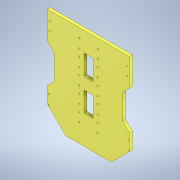
# Autodesk Inventor part: BaseCarro
Saved by Autodesk Inventor 2021 (Build 250183000, 183)
## iProperties
Created: 2021-02-05
Part Number: BaseCarro
Material: Plástico ABS
Document SubType Name: Modeling
Designer: jaime
Density: 1.06 g/cm^3
Appearance: Suave - Amarillo
Author: jaime
Autodesk Inventor part; units mm, degrees
ref_plane "YZ Plane" through (0, 0, 0) normal (1, 0, 0) x (0, 1, 0)
ref_plane "XZ Plane" through (0, 0, 0) normal (0, 1, 0) x (-1, 0, 0)
ref_plane "XY Plane" through (0, 0, 0) normal (0, 0, 1) x (1, 0, 0)
sketch "Boceto1" plane through (0, 0, 0) normal (0, 0, 1) x (1, 0, 0)
  line L0 (0, 0) -> (-180, 0)
  line L1 (-180, 0) -> (-180, -120)
  line L2 (-180, -120) -> (-150, -150)
  line L3 (-150, -150) -> (-150, -260)
  line L4 (-150, -260) -> (-180, -290)
  line L5 (-180, -290) -> (-180, -360)
  line L6 (-180, -360) -> (-100, -440)
  line L7 (-100, -440) -> (0, -440)
  line L8 (0, -440) -> (0, 0) construction
  line L9 (0, 0) -> (180, 0)
  line L10 (180, 0) -> (180, -120)
  line L11 (180, -120) -> (150, -150)
  line L12 (150, -150) -> (150, -260)
  line L13 (150, -260) -> (180, -290)
  line L14 (180, -290) -> (180, -360)
  line L15 (180, -360) -> (100, -440)
  line L16 (100, -440) -> (0, -440)
  dimension "d0" = 120
  dimension "d1" = 70
  dimension "d2" = 110
  dimension "d3" = 180
  dimension "d8" = 100
  dimension "d9" = 80
  dimension "d13" = 150
  dimension "d17" = 80
  dimension "d18" = 30
  dimension "d19" = 30
  constraints: 34 end point, 7 symmetric about line, 2 horizontal, 2 perpendicular, 1 parallel, 1 vertical
  measures "d0" distance of L0.end L1.end
  measures "d1" distance of L4.end L5.end
  measures "d2" distance of L2.end L3.end
  measures "d3" distance of L0.start L0.end
  measures "d8" distance of L6.end L7.end
  measures "d9" horizontal distance of L5.end L6.end
  measures "d13" distance between parallel lines of L3 L8
  measures "d17" horizontal distance of L5.end L6.end
  measures "d18" horizontal distance of L3.end L4.end
  measures "d19" horizontal distance of L1.end L2.end
extrude "Extrusión1" add sketch "Boceto1" along normal mid plane 12.55
sketch "Boceto2" plane through (0, 0, 6.275) normal (0, 0, 1) x (1, 0, 0)
  line L0 (0, 0) -> (0, -440)
  line L1 (-100, -440) -> (100, -440) projected
  line L2 (180, 0) -> (180, -120) projected
  line L3 (180, -120) -> (-179.9429, -120)
  line L4 (180, -120) -> (150, -150) projected
  line L5 (180, -120) -> (180, -60)
  line L6 (180, -60) -> (0, -60)
  line L7 (0, -60) -> (15, -60)
  line L8 (15, -60) -> (-15, -60)
  line L9 (180, -60) -> (170, -60)
  line L10 (170, -60) -> (170, -79.5)
  line L11 (170, -79.5) -> (170, -40.5)
  circle A0 centre (170, -40.5) radius 2.5
  circle A1 centre (170, -79.5) radius 2.5
  circle A2 centre (-170, -40.5) radius 2.5
  circle A3 centre (-170, -79.5) radius 2.5
  dimension "d20" = 60
  dimension "d22" = 30
  dimension "d23" = 10
  dimension "d25" = 39
  dimension "d26" = 5
  constraints: 18 end point, 5 point on line, 4 centre point, 3 symmetric about line, 2 midpoint, 2 perpendicular, 1 coincident, 1 horizontal, 3 other
  measures "d20" distance of L2.end L5.end
  measures "d22" distance of L7.end L8.end
  measures "d23" distance of L5.end L9.end
  measures "d25" distance of L10.end L11.end
  measures "d26" diameter of A0
extrude "Extrusión2" cut sketch "Boceto2" against normal blind 14.75 contours A0 | A1 | A2 | A3
sketch "Boceto3" plane through (0, 0, 6.275) normal (0, 0, 1) x (1, 0, 0)
  circle A0 centre (170, -40.5) radius 2.5 projected
  line L0 (170, -40.5) -> (170, -60)
  line L1 (170, -60) -> (0, -60)
  line L2 (0, -60) -> (0, -130)
  line L3 (0, -130) -> (40, -130)
  line L4 (40, -130) -> (-40, -130)
  line L5 (40, -130) -> (40, -110.5)
  circle A1 centre (40, -110.5) radius 2.5
  circle A2 centre (40, -149.5) radius 2.5
  circle A3 centre (-40, -110.5) radius 2.5
  circle A4 centre (-40, -149.5) radius 2.5
  line L6 (40, -130) -> (40, -200)
  line L7 (40, -200) -> (40, -165)
  line L8 (40, -165) -> (-88.7042, -165)
  circle A5 centre (40, -219.5) radius 2.5
  circle A6 centre (40, -180.5) radius 2.5
  circle A7 centre (-40, -219.5) radius 2.5
  circle A8 centre (-40, -180.5) radius 2.5
  line L9 (40, -180.5) -> (40, -200)
  line L10 (40, -200) -> (40, -270)
  line L11 (40, -270) -> (-42.5, -270)
  line L12 (40, -270) -> (40, -235)
  line L13 (40, -235) -> (-24.3521, -235)
  circle A9 centre (40, -359.5) radius 2.5
  circle A10 centre (40, -320.5) radius 2.5
  circle A11 centre (-40, -359.5) radius 2.5
  circle A12 centre (-40, -320.5) radius 2.5
  circle A13 centre (40, -250.5) radius 2.5
  circle A14 centre (40, -289.5) radius 2.5
  circle A15 centre (-40, -250.5) radius 2.5
  circle A16 centre (-40, -289.5) radius 2.5
  line L14 (40, -165) -> (40, -95)
  line L15 (40, -95) -> (-4.3592, -95)
  circle A17 centre (40, -79.5) radius 2.5
  circle A18 centre (40, -40.5) radius 2.5
  circle A19 centre (-40, -79.5) radius 2.5
  circle A20 centre (-40, -40.5) radius 2.5
  point P0 (0, 0)
  dimension "d29" = 19.5
  dimension "d30" = 70
  dimension "d31" = 40
  dimension "d32" = 80
  dimension "d33" = 19.5
  dimension "d34" = 5
  dimension "d37" = 70
  dimension "d38" = 70
  dimension "d39" = 35
  dimension "d46" = 70
  constraints: 32 end point, 20 centre point, 19 symmetric about line, 5 perpendicular, 5 vertical, 2 horizontal, 2 midpoint, 2 point on line, 1 coincident, 19 other
  measures "d29" distance of L0.start L0.end
  measures "d30" distance of L1.end L2.end
  measures "d31" distance of L2.end L3.end
  measures "d32" distance of L3.end L4.end
  measures "d33" distance of L3.end L5.end
  measures "d34" diameter of A1
  measures "d37" distance of L3.end L6.end
  measures "d38" distance of L6.end L10.end
  measures "d39" distance of L10.end L12.end
  measures "d46" distance of L7.end L14.end
extrude "Extrusión3" cut sketch "Boceto3" against normal blind 14.75 contours L14 L5 A1 | A1 L5 L14 | A2 L6 | L6 A2 | A3 | A4 | A6 L6 | L6 A6 | A5 L10 | L10 A5 | A7 | A8 | A13 L10 | L10 A13 | A9 | A10 | A11 | A12 | A14 | A15 | A16 | A17 | A18 | A19 | A20
sketch "Boceto4" plane through (0, 0, 6.275) normal (0, 0, 1) x (1, 0, 0)
  circle A0 centre (40, -320.5) radius 2.5 projected
  line L0 (40, -320.5) -> (180, -320.5)
  line L1 (180, -360) -> (180, -290) projected
  line L2 (180, -320.5) -> (175, -320.5)
  line L3 (175, -320.5) -> (175, -359.5)
  circle A1 centre (175, -320.5) radius 2.5
  circle A2 centre (175, -359.5) radius 2.5
  line L4 (-100, -440) -> (100, -440) projected
  line L5 (0, -440) -> (0, 0)
  circle A3 centre (-175, -320.5) radius 2.5
  circle A4 centre (-175, -359.5) radius 2.5
  dimension "d40" = 5
  dimension "d41" = 39
  dimension "d42" = 5
  dimension "d43" = 5
  constraints: 8 end point, 4 centre point, 2 coincident, 2 point on line, 2 symmetric about line, 1 horizontal, 1 midpoint, 1 perpendicular, 1 vertical, 2 other
  measures "d40" distance of L0.end L2.end
  measures "d41" distance of L2.end L3.end
  measures "d42" diameter of A1
  measures "d43" diameter of A2
extrude "Extrusión4" cut sketch "Boceto4" against normal blind 14.75 contours L0 A1 | L3 A1 L0 | L0 A1 L3 | A2 | A3 | A4
sketch "Boceto6" plane through (0, 0, -6.275) normal (0, 0, -1) x (-1, 0, 0)
  circle A0 centre (40, -289.5) radius 2.5 projected
  circle A1 centre (-40, -289.5) radius 2.5 projected
  line L0 (40, -289.5) -> (-40, -289.5)
  circle A2 centre (-40, -250.5) radius 2.5 projected
  line L1 (-40, -289.5) -> (-40, -250.5)
  circle A3 centre (40, -250.5) radius 2.5 projected
  line L2 (-40, -250.5) -> (40, -250.5)
  line L3 (40, -250.5) -> (40, -289.5)
  line L4 (0, -289.5) -> (20, -289.5)
  line L5 (20, -289.5) -> (20, -250.5)
  line L6 (20, -250.5) -> (-20, -250.5)
  line L7 (-20, -250.5) -> (-20, -289.5)
  line L8 (20, -289.5) -> (20, -314.5)
  line L9 (20, -314.5) -> (-20, -314.5)
  line L10 (-20, -314.5) -> (-20, -289.5)
  line L11 (20, -250.5) -> (20, -225.5)
  line L12 (20, -225.5) -> (-20, -225.5)
  line L13 (-20, -225.5) -> (-20, -250.5)
  point P0 (0, 0)
  dimension "d56" = 40
  dimension "d57" = 25
  dimension "d58" = 25
  constraints: 28 end point, 10 perpendicular, 6 point on line, 1 horizontal, 1 midpoint
  measures "d56" distance of L5.end L6.end
  measures "d57" distance of L4.end L8.end
  measures "d58" distance of L5.end L11.end
extrude "Extrusión6" cut sketch "Boceto6" against normal blind 14.75 contours L8 L9 L10 L0 | L0 L7 L2 L5 | L2 L13 L12 L11
sketch "Boceto7" plane through (0, 0, -6.275) normal (0, 0, -1) x (-1, 0, 0)
  circle A0 centre (40, -110.5) radius 2.5 projected
  circle A1 centre (-40, -110.5) radius 2.5 projected
  line L0 (40, -110.5) -> (-40, -110.5)
  circle A2 centre (-40, -149.5) radius 2.5 projected
  line L1 (-40, -110.5) -> (-40, -149.5)
  line L2 (-40, -149.5) -> (40, -149.5)
  line L3 (40, -149.5) -> (40, -110.5)
  line L4 (0, -149.5) -> (-20, -149.5)
  line L5 (-20, -149.5) -> (20, -149.5)
  line L6 (20, -149.5) -> (20, -110.5)
  line L7 (20, -149.5) -> (20, -174.5)
  line L8 (20, -174.5) -> (-20, -174.5)
  line L9 (-20, -174.5) -> (-20, -149.5)
  line L10 (20, -110.5) -> (20, -85.5)
  line L11 (20, -85.5) -> (-20, -85.5)
  line L12 (-20, -85.5) -> (-20, -110.5)
  line L13 (-20, -149.5) -> (-20, -110.5)
  point P0 (0, 0)
  dimension "d63" = 25
  dimension "d64" = 40
  dimension "d65" = 25
  dimension "d66" = 40
  constraints: 28 end point, 7 perpendicular, 4 point on line, 2 horizontal, 1 collinear, 1 midpoint, 1 vertical
  measures "d63" distance of L5.end L7.end
  measures "d64" distance of L7.end L8.end
  measures "d65" distance of L6.end L10.end
  measures "d66" distance of L10.end L11.end
extrude "Extrusión7" cut sketch "Boceto7" against normal blind 14.75 contours L6 L2 L13 L0 | L0 L12 L11 L10 | L7 L8 L9 L2
sketch "Boceto8" plane through (0, 0, -6.275) normal (0, 0, -1) x (-1, 0, 0)
  line L0 (0, 0) -> (0, -20)
  line L1 (0, -20) -> (-45, -20)
  line L2 (-45, -20) -> (45, -20)
  line L3 (45, -20) -> (45, -30)
  line L4 (45, -30) -> (55, -30)
  line L5 (55, -30) -> (55, -20)
  line L6 (55, -20) -> (45, -20)
  line L7 (-45, -20) -> (-45, -30)
  line L8 (-45, -30) -> (-55, -30)
  line L9 (-55, -30) -> (-55, -20)
  line L10 (-55, -20) -> (-45, -20)
  line L11 (55, -30) -> (55, -115)
  line L12 (55, -115) -> (45, -115)
  line L13 (45, -115) -> (45, -125)
  line L14 (45, -125) -> (55, -125)
  line L15 (55, -125) -> (55, -115)
  line L16 (-45, -30) -> (-45, -115)
  line L17 (-45, -115) -> (-55, -115)
  line L18 (-55, -115) -> (-55, -125)
  line L19 (-55, -125) -> (-45, -125)
  line L20 (-45, -125) -> (-45, -115)
  dimension "d69" = 20
  dimension "d70" = 45
  dimension "d71" = 90
  dimension "d72" = 10
  dimension "d73" = 10
  dimension "d74" = 10
  dimension "d75" = 10
  dimension "d76" = 10
  dimension "d77" = 10
  dimension "d78" = 85
  dimension "d79" = 10
  dimension "d80" = 10
  dimension "d81" = 10
  dimension "d82" = 85
  dimension "d83" = 10
  dimension "d84" = 10
  dimension "d85" = 10
  constraints: 42 end point, 8 perpendicular, 7 point on line, 3 vertical
  measures "d69" distance of L0.start L0.end
  measures "d70" distance of L0.end L1.end
  measures "d71" distance of L1.end L2.end
  measures "d72" distance of L2.end L3.end
  measures "d73" distance of L3.end L4.end
  measures "d74" distance of L4.end L5.end
  measures "d75" distance of L1.end L7.end
  measures "d76" distance of L7.end L8.end
  measures "d77" distance of L8.end L9.end
  measures "d78" distance of L4.end L11.end
  measures "d79" distance of L11.end L12.end
  measures "d80" distance of L12.end L13.end
  measures "d81" distance of L13.end L14.end
  measures "d82" distance of L7.end L16.end
  measures "d83" distance of L16.end L17.end
  measures "d84" distance of L17.end L18.end
  measures "d85" distance of L18.end L19.end
extrude "Extrusión8" cut sketch "Boceto8" against normal blind 7
